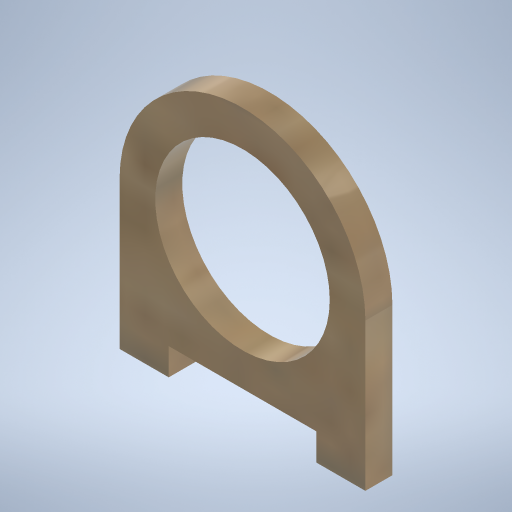
# Autodesk Inventor part: motor_setter_middle
Saved by Autodesk Inventor 2024.1 (Build 281209000, 209)
## iProperties
Created: 2025-10-20
Part Number: motor_setter_middle
Material: 木材 (カエデ材)
Document SubType Name: Modeling
Designer: hibik
Density: 0.67 g/cm^3
Appearance: ナチュラル カエデ材 - 光沢 濃い着色
Author: hibik
Autodesk Inventor part; units mm, degrees
ref_plane "YZ Plane" through (0, 0, 0) normal (1, 0, 0) x (0, 1, 0)
ref_plane "XZ Plane" through (0, 0, 0) normal (0, 1, 0) x (-1, 0, 0)
ref_plane "XY Plane" through (0, 0, 0) normal (0, 0, 1) x (1, 0, 0)
sketch "スケッチ1" plane through (0, 0, 0) normal (0, 0, 1) x (1, 0, 0)
  circle A0 centre (0, 0) radius 17.75
  line L0 (-25, 30.5) -> (25, 30.5)
  line L1 (25, 30.5) -> (25, -24.5)
  line L2 (25, -24.5) -> (-25, -24.5)
  line L3 (-25, -24.5) -> (-25, 30.5)
  line L4 (-25, -24.5) -> (-15, -24.5)
  line L5 (-15, -24.5) -> (-15, -30)
  line L6 (-15, -30) -> (-25, -30)
  line L7 (-25, -30) -> (-25, -24.5)
  line L8 (15, -24.5) -> (25, -24.5)
  line L9 (25, -24.5) -> (25, -30)
  line L10 (25, -30) -> (15, -30)
  line L11 (15, -30) -> (15, -24.5)
  circle A1 centre (0, 0) radius 25
  point P0 (0, 30.5)
  point P1 (-15, -24.5)
  point P2 (-25, 0)
  point P3 (25, 0)
  dimension "d0" = 35.5
  dimension "d1" = 24.5
  dimension "d2" = 50
  dimension "d3" = 55
  dimension "d6" = 5.5
  dimension "d7" = 10
  constraints: 24 end point, 6 parallel, 3 collinear, 3 horizontal, 3 perpendicular, 2 centre point, 2 coincident, 1 midpoint, 1 point on line, 1 tangent, 1 vertical alignment
  measures "d0" diameter of A0
  measures "d1" distance from line of L2 point (0, 0)
  measures "d2" distance of L0.start L0.end
  measures "d3" distance of L2.end L0.start
  measures "d6" distance of L6.end L2.end
  measures "d7" distance of L5.end L6.end
extrude "押し出し1" add sketch "スケッチ1" along normal blind 5.5 contours A1 L2 L3 | A1 L2 | L1 L2 A1 | L2 L5 L6 L7 | L9 L10 L11 L2 picked at (-0.7132, -22.2069)
